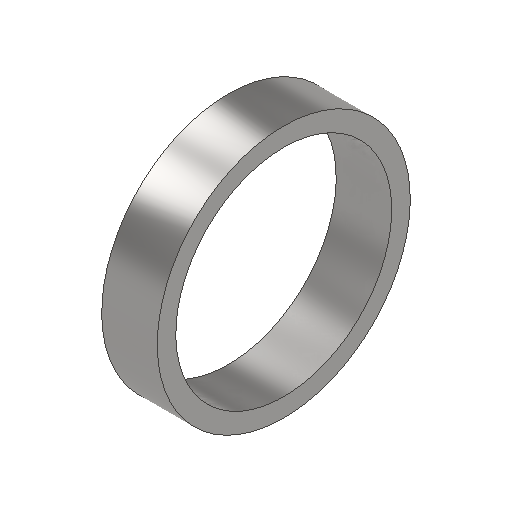
# Autodesk Inventor part: Part2
Saved by Autodesk Inventor 2024.2 (Build 282272000, 272)
## iProperties
Created: 2019-06-28
Part Number: Part2
Material: Stainless Steel
Document SubType Name: Modeling
Designer: Nakamura
Density: 8 g/cm^3
Appearance: Semi-Polished
Mass: 1.65032 g
Surface Area: 4.58421 cm^2
Volume: 0.20629 cm^3
Author: Nakamura
Autodesk Inventor part; units mm, degrees
ref_plane "YZ Plane" through (0, 0, 0) normal (1, 0, 0) x (0, 1, 0)
ref_plane "XZ Plane" through (0, 0, 0) normal (0, 1, 0) x (-1, 0, 0)
ref_plane "XY Plane" through (0, 0, 0) normal (0, 0, 1) x (1, 0, 0)
sketch "スケッチ1" plane through (0, 0, 0) normal (0, 0, 1) x (1, 0, 0)
  line L0 (-3.6, 8.2) -> (0, 8.2)
  line L1 (0, 8.2) -> (0, 7)
  line L2 (0, 7) -> (-3.6, 7)
  line L3 (-3.6, 7) -> (-3.6, 8.2)
  line L4 (-16.7746, 0) -> (0, 0)
  dimension "d1" = 3.6
  dimension "d2" = 1.2
  dimension "d4" = 14
  constraints: 10 end point, 3 perpendicular, 1 point on line, 1 vertical
  measures "d1" distance of L0.start L0.end
  measures "d2" distance of L0.end L1.end
  measures "d4" diameter of L2 L4
revolve "回転1" add sketch "スケッチ1" angle 360 about axis through (-16.7746, 0, 0) along (1, 0, 0)
